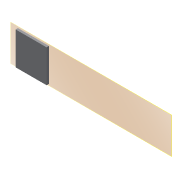
# Autodesk Inventor part: BallCasterMountFlat
Saved by Autodesk Inventor 2018 (Build 220112000, 112)
## iProperties
Created: 2019-02-16
Part Number: BallCasterMountFlat
Material: Generic
Document SubType Name: Modeling
Designer: ball
Density: 1 g/cm^3
Appearance: Default
Author: ball
Autodesk Inventor part; units mm, degrees
ref_plane "YZ Plane" through (0, 0, 0) normal (1, 0, 0) x (0, 1, 0)
ref_plane "XZ Plane" through (0, 0, 0) normal (0, 1, 0) x (-1, 0, 0)
ref_plane "XY Plane" through (0, 0, 0) normal (0, 0, 1) x (1, 0, 0)
ref_plane "Work Plane1" through (0, 0, 0) normal (0, 0, 1) x (1, 0, 0)
sketch "Sketch1" plane through (0, 0, 0) normal (0, 0, 1) x (1, 0, 0)
  line L0 (-192, 0) -> (0, 0) construction
  line L1 (-192, 0) -> (-192, -43) construction
  line L2 (-192, -43) -> (0, -43) construction
  line L3 (-192, -43) -> (-151.3614, -43)
  line L4 (-151.3614, -43) -> (-151.3614, 0)
  line L5 (-151.3614, 0) -> (-192, 0)
  line L6 (-192, 0) -> (-192, -43)
  constraints: 8 end point, 2 parallel, 1 horizontal, 1 perpendicular, 1 point on line
extrude "Extrusion1" add sketch "Sketch1" along normal blind 3.048
body "Solid1"
